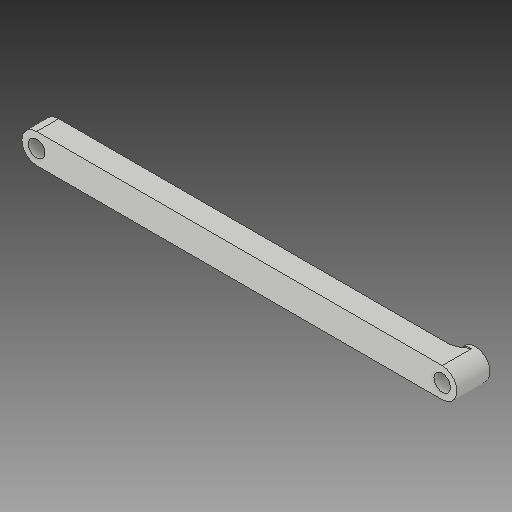
# Autodesk Inventor part: 110_single
Saved by Autodesk Inventor 2017 (Build 210142000, 142)
## iProperties
Created: 2020-03-22
Part Number: 110_single
Material: Generic
Document SubType Name: Modeling
Designer: LaNave
Density: 1 g/cm^3
Appearance: Default
Mass: 2.26689 g
Surface Area: 24.3723 cm^2
Volume: 2.26689 cm^3
Author: LaNave
Autodesk Inventor part; units mm, degrees
ref_plane "YZ Plane" through (0, 0, 0) normal (1, 0, 0) x (0, 1, 0)
ref_plane "XZ Plane" through (0, 0, 0) normal (0, 1, 0) x (-1, 0, 0)
ref_plane "XY Plane" through (0, 0, 0) normal (0, 0, 1) x (1, 0, 0)
sketch "Sketch1" plane through (0, 0, 0) normal (0, 0, 1) x (1, 0, 0)
  circle A0 centre (0, 0) radius 2.25
  circle A1 centre (-110, 0) radius 2.25
  line L0 (-2.3539, -2.2409) -> (0, 0)
  line L1 (0, 0) -> (-110, 0) construction
  line L2 (0, 4) -> (-110, 4)
  line L3 (-110, -4) -> (0, -4)
  arc A2 (0, -4) -> (0, 4) centre (0, 0) ccw
  arc A3 (-110, 4) -> (-110, -4) centre (-110, 0) ccw
  point P0 (-55, 0)
  dimension "d1" = 4.5
  dimension "d17" = 4.5
  dimension "d29" = 8
  constraints: 10 end point, 4 centre point, 4 point on circle, 4 tangent, 2 coincident, 1 horizontal, 1 midpoint, 1 parallel
  measures "d1" diameter of A0
  measures "d17" diameter of A1
  measures "d29" diameter of A3
extrude "Extrusion1" add sketch "Sketch1" along normal blind 6
sketch "Sketch2" plane through (0, 0, 0) normal (0, 0, -1) x (-1, 0, 0)
  circle A0 centre (0, 0) radius 2.25
  circle A1 centre (110, 0) radius 2.25 projected
  circle A2 centre (110, 0) radius 2.25
  circle A3 centre (0, 0) radius 2.25 projected
  circle A4 centre (0, 0) radius 4
  circle A5 centre (110, 0) radius 4
  dimension "d23" = 4.5
  dimension "d24" = 4.5
  dimension "d26" = 8
  dimension "d27" = 8
  constraints: 4 centre point, 3 coincident
  measures "d23" diameter of A2
  measures "d24" diameter of A0
  measures "d26" diameter of A4
  measures "d27" diameter of A5
extrude "Extrusion2" add sketch "Sketch2" along normal blind 3 contours A4
fillet "Fillet4" radius 2 2 edges at (-2.8284, 2.8284, 0) (-2.8284, -2.8284, 0)
scale "Scale1" factors (0.5, 0.5, 0.5) then translate (-27.5, 2, 3) bodies 1
body "Solid1"
